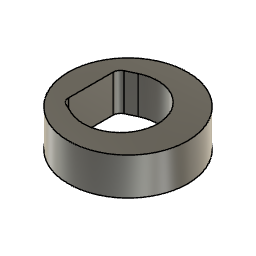
Eccentric Nut (Autodesk Fusion 360 design; units mm, degrees)
Autodesk Fusion 360 part; units mm, degrees
sketch "Sketch1" plane through (0, 0, 0) normal (0, 0, 1) x (1, 0, 0)
  circle A0 centre (0, 0) radius 4
  circle A1 centre (-0.5, 0) radius 2.5
  line L0 (-2.5, 1.5) -> (-2.5, -1.5)
  circle A2 centre (-2, 1.5) radius 0.5
  line L1 (-2.8087, 1.6679) -> (-0.6979, 2.676)
  line L2 (-0.5, 0) -> (0, 0)
  line L3 (-2.8087, -1.6679) -> (-0.6979, -2.676)
  circle A3 centre (-2, -1.5) radius 0.5
  dimension "d1" = 8
  dimension "d2" = 5
  dimension "d3" = 0.5
  dimension "d4" = 2
  dimension "d13" = 1
  constraint coincident A0.centre L2.end
  constraint horizontal A0.centre A1.centre
  constraint vertical L0
  constraint coincident A1 L0.start
  constraint coincident A1 L0.end
  constraint horizontal A2.centre L0.start
  constraint tangent L0 A2
  constraint tangent A1 L1
  constraint tangent A2 L1
  constraint coincident A1.centre L2.start
  constraint symmetric A2 L2 A3
  constraint symmetric L1.start L2 L3.start
  constraint symmetric L1.end L2 L3.end
  measures "d1" diameter of A0
  measures "d2" diameter of A1
  measures "d3" distance of A0.centre A1.centre
  measures "d4" distance of A1.centre L0
  measures "d13" diameter of A2
extrude "Extrude3" add sketch "Sketch1" along normal blind 2.5 contours A0 | A1 L0
